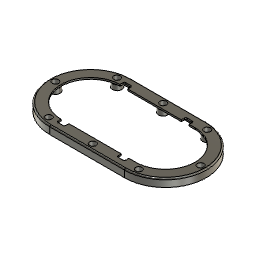
LG portable AC adapter (Autodesk Fusion 360 design; units mm, degrees)
Autodesk Fusion 360 part; units mm, degrees
sketch "Sketch1" plane through (0, 0, 0) normal (0, 0, 1) x (1, 0, 0)
  line L0 (0, 0) -> (210, 0)
  line L1 (210, 0) -> (210, 93)
  line L2 (210, 93) -> (0, 93)
  line L3 (0, 93) -> (0, 0)
  circle A0 centre (46.5, 46.5) radius 46.5
  circle A1 centre (163.5, 46.5) radius 46.5
  line L4 (47, 0) -> (59, 0)
  line L5 (59, 0) -> (59, -7)
  line L6 (59, -7) -> (47, -7)
  line L7 (47, -7) -> (47, 0)
  line L8 (46, 93) -> (58, 93)
  line L9 (58, 93) -> (58, 100)
  line L10 (58, 100) -> (46, 100)
  line L11 (46, 100) -> (46, 93)
  line L12 (154, 93) -> (142, 93)
  line L13 (142, 93) -> (142, 100)
  line L14 (142, 100) -> (154, 100)
  line L15 (154, 100) -> (154, 93)
  line L16 (141, 0) -> (153, 0)
  line L17 (153, 0) -> (153, -7)
  line L18 (153, -7) -> (141, -7)
  line L19 (141, -7) -> (141, 0)
  line L20 (-15, -15) -> (225, -15)
  line L21 (225, -15) -> (225, 108)
  line L22 (225, 108) -> (-15, 108)
  line L23 (-15, 108) -> (-15, -15)
  circle A2 centre (46.5, 46.5) radius 61.5
  circle A3 centre (163.5, 46.5) radius 61.5
  dimension "d1" = 210
  dimension "d2" = 93
  dimension "d3" = 47
  dimension "d4" = 12
  dimension "d6" = 46
  dimension "d7" = 12
  dimension "d9" = 56
  dimension "d10" = 12
  dimension "d12" = 57
  dimension "d13" = 12
  dimension "d15" = 15
  dimension "d16" = 15
  dimension "d17" = 15
  dimension "d18" = 7
  dimension "d19" = 7
  dimension "d20" = 7
  dimension "d21" = 7
  constraint horizontal L0
  constraint vertical L1
  constraint horizontal L2
  constraint vertical L3
  constraint coincident L0.start L3.end
  constraint tangent L0 A0
  constraint tangent L0 A1
  constraint tangent L2 A1
  constraint tangent L1 A1
  constraint tangent L2 A0
  constraint tangent L3 A0
  constraint horizontal L4
  constraint vertical L5
  constraint horizontal L6
  constraint vertical L7
  constraint coincident L0 L4.start
  constraint horizontal L8
  constraint vertical L9
  constraint horizontal L10
  constraint vertical L11
  constraint coincident L2 L8.start
  constraint horizontal L12
  constraint vertical L13
  constraint horizontal L14
  constraint vertical L15
  constraint coincident L2 L12.start
  constraint horizontal L16
  constraint vertical L17
  constraint horizontal L18
  constraint vertical L19
  constraint coincident L0 L16.start
  measures "d1" distance of L1.end L2.end
  measures "d2" distance of L0.end L1.end
  measures "d3" distance of L3 L7
  measures "d4" distance of L5.end L6.end
  measures "d6" distance of L3 L11
  measures "d7" distance of L9.end L10.end
  measures "d9" distance of L1 L15
  measures "d10" distance of L13 L15
  measures "d12" distance of L1 L17
  measures "d13" distance of L17.end L18.end
  measures "d18" distance of L2 L10
  measures "d19" distance of L2 L14
  measures "d20" distance of L0 L6
  measures "d21" distance of L0 L18
extrude "Extrude1" add sketch "Sketch1" along normal blind 2.4 contours L0 L5 L6 L7 A2 | L0 L3 A0 A2 | L0 L20 A2 A3 | L3 A2 | L2 L3 A0 L8 A2 | L0 L17 L18 L19 A3 | L2 L9 L10 L11 A2 | L0 L1 A1 A3 | L2 L22 A2 A3 | L2 L13 L14 L15 A3 | L1 A3 | L1 L2 A1 A3
ref_plane "WorkPlane1" through (105, 100.5, -10) normal (0, 0, 1) x (1, 0, 0)
sketch "Sketch2" plane through (0, 0, -10) normal (0, 0, 1) x (1, 0, 0)
  line L0 (153, 0) -> (163.5, 0)
  arc A0 (163.5, 0) -> (163.5, 93) centre (163.5, 46.5) ccw
  line L1 (163.5, 93) -> (154, 93)
  line L2 (154, 93) -> (154, 100)
  line L3 (154, 100) -> (142, 100)
  line L4 (142, 100) -> (142, 93)
  line L5 (142, 93) -> (58, 93)
  line L6 (58, 93) -> (58, 100)
  line L7 (58, 100) -> (46, 100)
  line L8 (46, 100) -> (46, 93)
  line L9 (46, 93) -> (46.5, 93)
  arc A1 (46.5, 93) -> (46.5, 0) centre (46.5, 46.5) ccw
  line L10 (46.5, 0) -> (47, 0)
  line L11 (47, 0) -> (47, -7)
  line L12 (47, -7) -> (59, -7)
  line L13 (59, -7) -> (59, 0)
  line L14 (59, 0) -> (141, 0)
  line L15 (141, 0) -> (141, -7)
  line L16 (141, -7) -> (153, -7)
  line L17 (153, -7) -> (153, 0)
  arc A2 (163.5, -15) -> (163.5, 108) centre (163.5, 46.5) ccw
  line L18 (163.5, -15) -> (46.5, -15)
  arc A3 (46.5, 108) -> (46.5, -15) centre (46.5, 46.5) ccw
  line L19 (46.5, 108) -> (163.5, 108)
  line L20 (163.5, -17.4) -> (46.5, -17.4)
  arc A4 (46.5, 110.4) -> (46.5, -17.4) centre (46.5, 46.5) ccw
  line L21 (46.5, 110.4) -> (163.5, 110.4)
  arc A5 (163.5, -17.4) -> (163.5, 110.4) centre (163.5, 46.5) ccw
  dimension "d25" = -2.4
extrude "Extrude2" add sketch "Sketch2" along normal up to surface (12.4 mm away) contours L20 A4 L21 A5
sketch "Sketch3" plane through (0, 0, 2.4) normal (0, 0, 1) x (-1, 0, 0)
  line L0 (-163.5, -110.4) -> (-46.5, -110.4)
  arc A0 (-46.5, -110.4) -> (-46.5, 17.4) centre (-46.5, -46.5) ccw
  line L1 (-46.5, 17.4) -> (-163.5, 17.4)
  arc A1 (-163.5, 17.4) -> (-163.5, -110.4) centre (-163.5, -46.5) ccw
  line L2 (-163.5, 0) -> (-153, 0)
  line L3 (-153, 0) -> (-153, 7)
  line L4 (-153, 7) -> (-141, 7)
  line L5 (-141, 7) -> (-141, 0)
  line L6 (-141, 0) -> (-59, 0)
  line L7 (-59, 0) -> (-59, 7)
  line L8 (-59, 7) -> (-47, 7)
  line L9 (-47, 7) -> (-47, 0)
  line L10 (-47, 0) -> (-46.5, 0)
  arc A2 (-46.5, -93) -> (-46.5, 0) centre (-46.5, -46.5) ccw
  line L11 (-46.5, -93) -> (-46, -93)
  line L12 (-46, -93) -> (-46, -100)
  line L13 (-46, -100) -> (-58, -100)
  line L14 (-58, -100) -> (-58, -93)
  line L15 (-58, -93) -> (-142, -93)
  line L16 (-142, -93) -> (-142, -100)
  line L17 (-142, -100) -> (-154, -100)
  line L18 (-154, -100) -> (-154, -93)
  line L19 (-154, -93) -> (-163.5, -93)
  arc A3 (-163.5, 0) -> (-163.5, -93) centre (-163.5, -46.5) ccw
  circle A4 centre (-218.5, -46.5) radius 5
  circle A5 centre (-218.5, -46.5) radius 7.4
  circle A6 centre (8.5, -46.5) radius 5
  circle A7 centre (8.5, -46.5) radius 7.4
  circle A8 centre (-105, -101.5) radius 5
  circle A9 centre (-105, -101.5) radius 7.4
  line L20 (-46.5, -46.5) -> (-163.5, -46.5) construction
  circle A10 centre (-105, 8.5) radius 5
  circle A11 centre (-105, 8.5) radius 7.4
  circle A12 centre (-175.5, -100) radius 5
  circle A13 centre (-175.5, -100) radius 7.4
  circle A14 centre (-175.5, 7) radius 7.4
  circle A15 centre (-175.5, 7) radius 5
  line L21 (-105, -101.5) -> (-105, 8.5) construction
  circle A16 centre (-34.5, -100) radius 5
  circle A17 centre (-34.5, -100) radius 7.4
  circle A18 centre (-34.5, 7) radius 5
  circle A19 centre (-34.5, 7) radius 7.4
  circle A20 centre (-34.5, -100) radius 2.1
  circle A21 centre (-105, -101.5) radius 2.1
  circle A22 centre (-175.5, -100) radius 2.1
  circle A23 centre (-34.5, 7) radius 2.1
  circle A24 centre (-105, 8.5) radius 2.1
  circle A25 centre (-175.5, 7) radius 2.1
  circle A26 centre (8.5, -46.5) radius 2.1
  circle A27 centre (-218.5, -46.5) radius 2.1
  point P0 (-105, -46.5)
  dimension "d28" = 10
  dimension "d29" = 2.4
  dimension "d30" = 55
  dimension "d31" = 10
  dimension "d32" = 2.4
  dimension "d33" = 55
  dimension "d34" = 10
  dimension "d35" = 2.4
  dimension "d36" = 55
  dimension "d37" = 2.4
  dimension "d38" = 10
  dimension "d39" = 55
  dimension "d42" = 2.4
  dimension "d43" = 10
  dimension "d44" = 53.5
  dimension "d45" = 12
  dimension "d46" = 4.2
  dimension "d47" = 4.2
  dimension "d48" = 4.2
  dimension "d49" = 4.2
  dimension "d50" = 4.2
  dimension "d51" = 4.2
  dimension "d52" = 4.2
  dimension "d53" = 4.2
  constraint horizontal A1.centre A4.centre
  constraint horizontal A0.centre A6.centre
  constraint coincident A0.centre A2.centre
  constraint coincident A1.centre A3.centre
  constraint midpoint L20 P0
  constraint vertical A8.centre P0
  constraint vertical P0 A10.centre
  constraint symmetric L20 A12 A15
  constraint symmetric L20 A13 A14
  constraint coincident A8.centre A9.centre
  constraint coincident A10.centre A11.centre
  constraint symmetric A12 L21 A16
  constraint symmetric A13 L21 A17
  constraint symmetric A14 L21 A19
  constraint symmetric A15 L21 A18
  constraint concentric A16 A20
  constraint concentric A8 A21
  constraint concentric A12 A22
  constraint concentric A19 A23
  constraint concentric A10 A24
  constraint concentric A15 A25
  constraint concentric A6 A26
  constraint concentric A4 A27
  measures "d28" diameter of A4
  measures "d30" distance of A1.centre A4.centre
  measures "d31" diameter of A6
  measures "d33" distance of A0.centre A6.centre
  measures "d34" diameter of A8
  measures "d36" distance of A8.centre L20
  measures "d38" diameter of A10
  measures "d39" distance of L20 A10.centre
  measures "d43" diameter of A12
  measures "d44" vertical distance of A1.centre A12.centre
  measures "d45" horizontal distance of A1.centre A12.centre
  measures "d46" diameter of A20
  measures "d47" diameter of A21
  measures "d48" diameter of A22
  measures "d49" diameter of A27
  measures "d50" diameter of A25
  measures "d51" diameter of A24
  measures "d52" diameter of A23
  measures "d53" diameter of A26
extrude "Extrude3" add sketch "Sketch3" against normal blind 12.4 contours A4 | A5 | A6 | A7 | A8 | A9 | A10 | A11 | A12 | A13 | A14 | A15 | A16 | A17 | A18 | A19 | A20 | A21 | A22 | A23 | A24 | A25 | A26 | A27
extrude "Extrude4" cut sketch "Sketch3" against normal blind 10 contours A4 | A6 | A8 | A10 | A12 | A15 | A16 | A18
extrude "Extrude5" cut sketch "Sketch3" against normal through all contours A20 | A21 | A22 | A23 | A24 | A25 | A26 | A27
fillet "Fillet1" radius 2 8 edges at (58, 100, 1.2) (46, 100, 1.2) (142, 100, 1.2) (154, 100, 1.2) (153, -7, 1.2) (141, -7, 1.2) (59, -7, 1.2) (47, -7, 1.2)
fillet "Fillet2" radius 2 20 edges at (173.8804, 92.7794, 0) (168.5826, 107.7896, 0) (136.0185, 108, 0) (105, 94.1, 0) (73.9815, 108, 0) (41.4174, 107.7896, 0) (211.4018, 85.0703, 0) (211.1, 46.5, 0) (211.4018, 7.9297, 0) (173.8804, 0.2206, 0) (136.0185, -15, 0) (168.5826, -14.7896, 0) (105, -1.1, 0) (41.4174, -14.7896, 0) (73.9815, -15, 0) (36.1196, 92.7794, 0) (-1.4018, 85.0703, 0) (-1.1, 46.5, 0) (-1.4018, 7.9297, 0) (36.1196, 0.2206, 0)
fillet "Fillet3" radius 2 4 edges at (227.4, 46.5, 2.4) (105, -17.4, 2.4) (-17.4, 46.5, 2.4) (105, 110.4, 2.4)
named bodies: "portable_ac_adapter"
